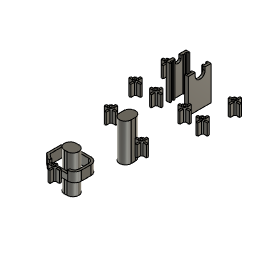
g304base (Autodesk Fusion 360 design; units mm, degrees)
Autodesk Fusion 360 part; units mm, degrees
note: some values were not read from the file. Set by a fixed rule: which sketch regions a step uses.
sketch "草图1" plane through (0, 0, 0) normal (0, 0, 1) x (1, 0, 0)
  circle A0 centre (-11.5, 1.7) radius 1.2
  circle A1 centre (-11.5, 1.7) radius 0.6
  circle A2 centre (11.6, -5.1) radius 0.6
  circle A3 centre (11.6, -5.1) radius 1.2
  circle A4 centre (7.5, 21.6) radius 0.6
  circle A5 centre (7.5, 21.6) radius 1.2
  circle A6 centre (-7.5, 21.6) radius 0.6
  circle A7 centre (-7.5, 21.6) radius 1.2
  circle A8 centre (-17.7, 38) radius 0.6
  circle A9 centre (-17.7, 38) radius 1.2
  circle A10 centre (-17.7, 20.9) radius 0.6
  circle A11 centre (-17.7, 20.9) radius 1.2
  circle A12 centre (17.7, 38) radius 0.6
  circle A13 centre (17.7, 38) radius 1.2
  circle A14 centre (17.7, 20.9) radius 0.6
  circle A15 centre (17.7, 20.9) radius 1.2
  circle A16 centre (0.3, -39.8) radius 0.6
  circle A17 centre (0.3, -39.8) radius 1.2
  dimension "d3" = 2.4
  dimension "d4" = 1.2
  dimension "d10" = 2.4
  dimension "d11" = 1.2
  dimension "d12" = 2.4
  dimension "d13" = 1.2
  dimension "d14" = 2.4
  dimension "d15" = 1.2
  dimension "d16" = 2.4
  dimension "d17" = 1.2
  dimension "d18" = 2.4
  dimension "d19" = 1.2
  dimension "d20" = 2.4
  dimension "d21" = 1.2
  dimension "d22" = 2.4
  dimension "d23" = 1.2
  dimension "d24" = 1.7
  dimension "d25" = 11.5
  dimension "d26" = 5.1
  dimension "d27" = 11.6
  dimension "d28" = 21.6
  dimension "d29" = 7.5
  dimension "d30" = 7.5
  dimension "d32" = 20.9
  dimension "d33" = 17.7
  dimension "d34" = 17.7
  dimension "d35" = 17.1
  dimension "d36" = 2.4
  dimension "d37" = 1.2
  dimension "d38" = 39.8
  dimension "d39" = 0.3
  constraint concentric A0 A1
  constraint concentric A2 A3
  constraint concentric A4 A5
  constraint concentric A6 A7
  constraint concentric A8 A9
  constraint concentric A10 A11
  constraint concentric A12 A13
  constraint concentric A14 A15
  constraint horizontal A4.centre A6.centre
  constraint horizontal A10.centre A14.centre
  constraint vertical A12.centre A14.centre
  constraint vertical A8.centre A10.centre
  constraint horizontal A8.centre A12.centre
  constraint concentric A16 A17
  measures "d3" diameter of A0
  measures "d4" diameter of A1
  measures "d10" diameter of A3
  measures "d11" diameter of A2
  measures "d12" diameter of A5
  measures "d13" diameter of A4
  measures "d14" diameter of A7
  measures "d15" diameter of A6
  measures "d16" diameter of A9
  measures "d17" diameter of A8
  measures "d18" diameter of A11
  measures "d19" diameter of A10
  measures "d20" diameter of A13
  measures "d21" diameter of A12
  measures "d22" diameter of A15
  measures "d23" diameter of A14
  measures "d24" vertical distance of origin A0.centre
  measures "d25" horizontal distance of origin A0.centre
  measures "d26" vertical distance of origin A2.centre
  measures "d27" horizontal distance of origin A2.centre
  measures "d28" vertical distance of origin A4.centre
  measures "d29" horizontal distance of origin A4.centre
  measures "d30" horizontal distance of origin A6.centre
  measures "d32" vertical distance of origin A14.centre
  measures "d33" horizontal distance of origin A14.centre
  measures "d34" horizontal distance of origin A10.centre
  measures "d35" vertical distance of A12.centre A14.centre
  measures "d36" diameter of A17
  measures "d37" diameter of A16
  measures "d38" vertical distance of origin A16.centre
  measures "d39" horizontal distance of origin A16.centre
sketch "草图2" plane through (0, 0, 0) normal (0, 0, 1) x (1, 0, 0)
  circle A0 centre (-11.5, 1.7) radius 1.2
  line L0 (-8.5, 2.2) -> (-14.5, 2.2)
  line L1 (-14.5, 2.2) -> (-14.5, 1.2)
  line L2 (-14.5, 1.2) -> (-8.5, 1.2)
  line L3 (-8.5, 1.2) -> (-8.5, 2.2)
  line L4 (-8.5, 2.2) -> (-14.5, 1.2) construction
  line L5 (-14.5, 2.2) -> (-8.5, 1.2) construction
  line L6 (-11, -1.3) -> (-12, -1.3)
  line L7 (-12, -1.3) -> (-12, 4.7)
  line L8 (-12, 4.7) -> (-11, 4.7)
  line L9 (-11, 4.7) -> (-11, -1.3)
  line L10 (-11, -1.3) -> (-12, 4.7) construction
  line L11 (-12, -1.3) -> (-11, 4.7) construction
  line L12 (11.1, -8.1) -> (11.1, -2.1)
  line L13 (12.1, -2.1) -> (12.1, -8.1)
  line L14 (14.6, -4.6) -> (8.6, -5.6) construction
  line L15 (14.6, -5.6) -> (14.6, -4.6)
  line L16 (11.1, -8.1) -> (12.1, -2.1) construction
  line L17 (8.6, -4.6) -> (14.6, -5.6) construction
  circle A1 centre (11.6, -5.1) radius 1.2
  line L18 (8.6, -5.6) -> (14.6, -5.6)
  line L19 (14.6, -4.6) -> (8.6, -4.6)
  line L20 (11.1, -2.1) -> (12.1, -2.1)
  line L21 (12.1, -8.1) -> (11.1, -8.1)
  line L22 (8.6, -4.6) -> (8.6, -5.6)
  line L23 (12.1, -8.1) -> (11.1, -2.1) construction
  line L24 (-18.2, 17.9) -> (-18.2, 23.9)
  line L25 (-17.2, 23.9) -> (-17.2, 17.9)
  line L26 (-14.7, 21.4) -> (-20.7, 20.4) construction
  line L27 (-14.7, 20.4) -> (-14.7, 21.4)
  line L28 (-18.2, 17.9) -> (-17.2, 23.9) construction
  line L29 (-20.7, 21.4) -> (-14.7, 20.4) construction
  circle A2 centre (-17.7, 20.9) radius 1.2
  line L30 (-20.7, 20.4) -> (-14.7, 20.4)
  line L31 (-14.7, 21.4) -> (-20.7, 21.4)
  line L32 (-18.2, 23.9) -> (-17.2, 23.9)
  line L33 (-17.2, 17.9) -> (-18.2, 17.9)
  line L34 (-20.7, 21.4) -> (-20.7, 20.4)
  line L35 (-17.2, 17.9) -> (-18.2, 23.9) construction
  line L36 (-8, 18.6) -> (-8, 24.6)
  line L37 (-7, 24.6) -> (-7, 18.6)
  line L38 (-4.5, 22.1) -> (-10.5, 21.1) construction
  line L39 (-4.5, 21.1) -> (-4.5, 22.1)
  line L40 (-8, 18.6) -> (-7, 24.6) construction
  line L41 (-10.5, 22.1) -> (-4.5, 21.1) construction
  circle A3 centre (-7.5, 21.6) radius 1.2
  line L42 (-10.5, 21.1) -> (-4.5, 21.1)
  line L43 (-4.5, 22.1) -> (-10.5, 22.1)
  line L44 (-8, 24.6) -> (-7, 24.6)
  line L45 (-7, 18.6) -> (-8, 18.6)
  line L46 (-10.5, 22.1) -> (-10.5, 21.1)
  line L47 (-7, 18.6) -> (-8, 24.6) construction
  line L48 (7, 18.6) -> (7, 24.6)
  line L49 (8, 24.6) -> (8, 18.6)
  line L50 (10.5, 22.1) -> (4.5, 21.1) construction
  line L51 (10.5, 21.1) -> (10.5, 22.1)
  line L52 (7, 18.6) -> (8, 24.6) construction
  line L53 (4.5, 22.1) -> (10.5, 21.1) construction
  circle A4 centre (7.5, 21.6) radius 1.2
  line L54 (4.5, 21.1) -> (10.5, 21.1)
  line L55 (10.5, 22.1) -> (4.5, 22.1)
  line L56 (7, 24.6) -> (8, 24.6)
  line L57 (8, 18.6) -> (7, 18.6)
  line L58 (4.5, 22.1) -> (4.5, 21.1)
  line L59 (8, 18.6) -> (7, 24.6) construction
  line L60 (17.2, 17.9) -> (17.2, 23.9)
  line L61 (18.2, 23.9) -> (18.2, 17.9)
  line L62 (20.7, 21.4) -> (14.7, 20.4) construction
  line L63 (20.7, 20.4) -> (20.7, 21.4)
  line L64 (17.2, 17.9) -> (18.2, 23.9) construction
  line L65 (14.7, 21.4) -> (20.7, 20.4) construction
  circle A5 centre (17.7, 20.9) radius 1.2
  line L66 (14.7, 20.4) -> (20.7, 20.4)
  line L67 (20.7, 21.4) -> (14.7, 21.4)
  line L68 (17.2, 23.9) -> (18.2, 23.9)
  line L69 (18.2, 17.9) -> (17.2, 17.9)
  line L70 (14.7, 21.4) -> (14.7, 20.4)
  line L71 (18.2, 17.9) -> (17.2, 23.9) construction
  line L72 (-18.2, 35) -> (-18.2, 41)
  line L73 (-17.2, 41) -> (-17.2, 35)
  line L74 (-14.7, 38.5) -> (-20.7, 37.5) construction
  line L75 (-14.7, 37.5) -> (-14.7, 38.5)
  line L76 (-18.2, 35) -> (-17.2, 41) construction
  line L77 (-20.7, 38.5) -> (-14.7, 37.5) construction
  circle A6 centre (-17.7, 38) radius 1.2
  line L78 (-20.7, 37.5) -> (-14.7, 37.5)
  line L79 (-14.7, 38.5) -> (-20.7, 38.5)
  line L80 (-18.2, 41) -> (-17.2, 41)
  line L81 (-17.2, 35) -> (-18.2, 35)
  line L82 (-20.7, 38.5) -> (-20.7, 37.5)
  line L83 (-17.2, 35) -> (-18.2, 41) construction
  line L84 (17.2, 35) -> (17.2, 41)
  line L85 (18.2, 41) -> (18.2, 35)
  line L86 (20.7, 38.5) -> (14.7, 37.5) construction
  line L87 (20.7, 37.5) -> (20.7, 38.5)
  line L88 (17.2, 35) -> (18.2, 41) construction
  line L89 (14.7, 38.5) -> (20.7, 37.5) construction
  circle A7 centre (17.7, 38) radius 1.2
  line L90 (14.7, 37.5) -> (20.7, 37.5)
  line L91 (20.7, 38.5) -> (14.7, 38.5)
  line L92 (17.2, 41) -> (18.2, 41)
  line L93 (18.2, 35) -> (17.2, 35)
  line L94 (14.7, 38.5) -> (14.7, 37.5)
  line L95 (18.2, 35) -> (17.2, 41) construction
  line L96 (-0.2, -42.8) -> (-0.2, -36.8)
  line L97 (0.8, -36.8) -> (0.8, -42.8)
  line L98 (3.3, -39.3) -> (-2.7, -40.3) construction
  line L99 (3.3, -40.3) -> (3.3, -39.3)
  line L100 (-0.2, -42.8) -> (0.8, -36.8) construction
  line L101 (-2.7, -39.3) -> (3.3, -40.3) construction
  circle A8 centre (0.3, -39.8) radius 1.2
  line L102 (-2.7, -40.3) -> (3.3, -40.3)
  line L103 (3.3, -39.3) -> (-2.7, -39.3)
  line L104 (-0.2, -36.8) -> (0.8, -36.8)
  line L105 (0.8, -42.8) -> (-0.2, -42.8)
  line L106 (-2.7, -39.3) -> (-2.7, -40.3)
  line L107 (0.8, -42.8) -> (-0.2, -36.8) construction
  point P0 (0.3, -39.8)
  point P1 (11.6, -5.1)
  point P2 (-11.5, 1.7)
  point P3 (-7.5, 21.6)
  point P4 (-17.7, 20.9)
  point P5 (7.5, 21.6)
  point P6 (17.7, 20.9)
  point P7 (17.7, 38)
  point P8 (-17.7, 38)
  point P9 (-11.5, 1.7)
  point P10 (-11.5, 1.7)
  point P11 (11.6, -5.1)
  point P12 (11.6, -5.1)
  point P13 (11.6, -5.1)
  point P14 (-17.7, 20.9)
  point P15 (-17.7, 20.9)
  point P16 (-17.7, 20.9)
  point P17 (-7.5, 21.6)
  point P18 (-7.5, 21.6)
  point P19 (-7.5, 21.6)
  point P20 (7.5, 21.6)
  point P21 (7.5, 21.6)
  point P22 (7.5, 21.6)
  point P23 (17.7, 20.9)
  point P24 (17.7, 20.9)
  point P25 (17.7, 20.9)
  point P26 (-17.7, 38)
  point P27 (-17.7, 38)
  point P28 (-17.7, 38)
  point P29 (17.7, 38)
  point P30 (17.7, 38)
  point P31 (17.7, 38)
  point P32 (0.3, -39.8)
  point P33 (0.3, -39.8)
  point P34 (0.3, -39.8)
  dimension "d42" = 2.4
  dimension "d43" = 6
  dimension "d44" = 1
  dimension "d45" = 1
  dimension "d46" = 6
  dimension "d47" = 2.4
  dimension "d48" = 6
  dimension "d49" = 1
  dimension "d50" = 1
  dimension "d51" = 6
  dimension "d52" = 2.4
  dimension "d53" = 6
  dimension "d54" = 1
  dimension "d55" = 1
  dimension "d56" = 6
  dimension "d57" = 2.4
  dimension "d58" = 6
  dimension "d59" = 1
  dimension "d60" = 1
  dimension "d61" = 6
  dimension "d62" = 2.4
  dimension "d63" = 6
  dimension "d64" = 1
  dimension "d65" = 1
  dimension "d66" = 6
  dimension "d67" = 2.4
  dimension "d68" = 6
  dimension "d69" = 1
  dimension "d70" = 1
  dimension "d71" = 6
  dimension "d72" = 2.4
  dimension "d73" = 6
  dimension "d74" = 1
  dimension "d75" = 1
  dimension "d76" = 6
  dimension "d77" = 2.4
  dimension "d78" = 6
  dimension "d79" = 1
  dimension "d80" = 1
  dimension "d81" = 6
  dimension "d82" = 2.4
  dimension "d83" = 6
  dimension "d84" = 1
  dimension "d85" = 1
  dimension "d86" = 6
  constraint coincident P9 P2
  constraint horizontal L0
  constraint perpendicular L0 L1
  constraint parallel L0 L2
  constraint parallel L1 L3
  constraint coincident L4 P10
  constraint coincident L5 P10
  constraint horizontal L6
  constraint perpendicular L6 L7
  constraint parallel L6 L8
  constraint parallel L7 L9
  constraint coincident L10 P10
  constraint coincident L11 P10
  constraint coincident P10 P9
  constraint coincident P13 P12
  constraint horizontal L19
  constraint perpendicular L19 L22
  constraint parallel L18 L19
  constraint parallel L15 L22
  constraint coincident P13 L14
  constraint coincident P13 L17
  constraint horizontal L21
  constraint perpendicular L12 L21
  constraint parallel L20 L21
  constraint parallel L12 L13
  constraint coincident P13 L23
  constraint coincident P13 L16
  constraint coincident P16 P15
  constraint horizontal L31
  constraint perpendicular L31 L34
  constraint parallel L30 L31
  constraint parallel L27 L34
  constraint coincident P16 L26
  constraint coincident P16 L29
  constraint horizontal L33
  constraint perpendicular L24 L33
  constraint parallel L32 L33
  constraint parallel L24 L25
  constraint coincident P16 L35
  constraint coincident P16 L28
  constraint coincident P19 P18
  constraint horizontal L43
  constraint perpendicular L43 L46
  constraint parallel L42 L43
  constraint parallel L39 L46
  constraint coincident P19 L38
  constraint coincident P19 L41
  constraint horizontal L45
  constraint perpendicular L36 L45
  constraint parallel L44 L45
  constraint parallel L36 L37
  constraint coincident P19 L47
  constraint coincident P19 L40
  constraint coincident P22 P21
  constraint horizontal L55
  constraint perpendicular L55 L58
  constraint parallel L54 L55
  constraint parallel L51 L58
  constraint coincident P22 L50
  constraint coincident P22 L53
  constraint horizontal L57
  constraint perpendicular L48 L57
  constraint parallel L56 L57
  constraint parallel L48 L49
  constraint coincident P22 L59
  constraint coincident P22 L52
  constraint coincident P25 P24
  constraint horizontal L67
  constraint perpendicular L67 L70
  constraint parallel L66 L67
  constraint parallel L63 L70
  constraint coincident P25 L62
  constraint coincident P25 L65
  constraint horizontal L69
  constraint perpendicular L60 L69
  constraint parallel L68 L69
  constraint parallel L60 L61
  constraint coincident P25 L71
  constraint coincident P25 L64
  constraint coincident P28 P27
  constraint horizontal L79
  constraint perpendicular L79 L82
  constraint parallel L78 L79
  constraint parallel L75 L82
  constraint coincident P28 L74
  constraint coincident P28 L77
  constraint horizontal L81
  constraint perpendicular L72 L81
  constraint parallel L80 L81
  constraint parallel L72 L73
  constraint coincident P28 L83
  constraint coincident P28 L76
  constraint coincident P31 P30
  constraint horizontal L91
  constraint perpendicular L91 L94
  constraint parallel L90 L91
  constraint parallel L87 L94
  constraint coincident P31 L86
  constraint coincident P31 L89
  constraint horizontal L93
  constraint perpendicular L84 L93
  constraint parallel L92 L93
  constraint parallel L84 L85
  constraint coincident P31 L95
  constraint coincident P31 L88
  constraint coincident P34 P33
  constraint horizontal L103
  constraint perpendicular L103 L106
  constraint parallel L102 L103
  constraint parallel L99 L106
  constraint coincident P34 L98
  constraint coincident P34 L101
  constraint horizontal L105
  constraint perpendicular L96 L105
  constraint parallel L104 L105
  constraint parallel L96 L97
  constraint coincident P34 L107
  constraint coincident P34 L100
  measures "d42" diameter of A0
  measures "d43" distance of L1.end L2.end
  measures "d44" distance of L0.end L1.end
  measures "d45" distance of L7.end L8.end
  measures "d46" distance of L6.end L7.end
  measures "d47" diameter of A1
  measures "d48" distance of L15.start L14.end
  measures "d49" distance of L14.end L17.start
  measures "d50" distance of L13.start L12.end
  measures "d51" distance of L12.start L12.end
  measures "d52" diameter of A2
  measures "d53" distance of L27.start L26.end
  measures "d54" distance of L26.end L29.start
  measures "d55" distance of L25.start L24.end
  measures "d56" distance of L24.start L24.end
  measures "d57" diameter of A3
  measures "d58" distance of L39.start L38.end
  measures "d59" distance of L38.end L41.start
  measures "d60" distance of L37.start L36.end
  measures "d61" distance of L36.start L36.end
  measures "d62" diameter of A4
  measures "d63" distance of L51.start L50.end
  measures "d64" distance of L50.end L53.start
  measures "d65" distance of L49.start L48.end
  measures "d66" distance of L48.start L48.end
  measures "d67" diameter of A5
  measures "d68" distance of L63.start L62.end
  measures "d69" distance of L62.end L65.start
  measures "d70" distance of L61.start L60.end
  measures "d71" distance of L60.start L60.end
  measures "d72" diameter of A6
  measures "d73" distance of L75.start L74.end
  measures "d74" distance of L74.end L77.start
  measures "d75" distance of L73.start L72.end
  measures "d76" distance of L72.start L72.end
  measures "d77" diameter of A7
  measures "d78" distance of L87.start L86.end
  measures "d79" distance of L86.end L89.start
  measures "d80" distance of L85.start L84.end
  measures "d81" distance of L84.start L84.end
  measures "d82" diameter of A8
  measures "d83" distance of L99.start L98.end
  measures "d84" distance of L98.end L101.start
  measures "d85" distance of L97.start L96.end
  measures "d86" distance of L96.start L96.end
sketch "草图3" plane through (0, 0, 0) normal (0, 0, 1) x (1, 0, 0)
  line L0 (19, 20) -> (16.4, 20)
  line L1 (16.4, 20) -> (16.4, 21.8)
  line L2 (16.4, 21.8) -> (19, 21.8)
  line L3 (19, 21.8) -> (19, 20)
  line L4 (19, 20) -> (16.4, 21.8) construction
  line L5 (16.4, 20) -> (19, 21.8) construction
  line L6 (16.4, 37.1) -> (19, 38.9) construction
  line L7 (19, 37.1) -> (16.4, 37.1)
  line L8 (19, 37.1) -> (16.4, 38.9) construction
  line L9 (16.4, 37.1) -> (16.4, 38.9)
  line L10 (16.4, 38.9) -> (19, 38.9)
  line L11 (19, 38.9) -> (19, 37.1)
  line L12 (-19, 37.1) -> (-16.4, 38.9) construction
  line L13 (-16.4, 37.1) -> (-19, 37.1)
  line L14 (-16.4, 37.1) -> (-19, 38.9) construction
  line L15 (-19, 37.1) -> (-19, 38.9)
  line L16 (-19, 38.9) -> (-16.4, 38.9)
  line L17 (-16.4, 38.9) -> (-16.4, 37.1)
  line L18 (-19, 20) -> (-16.4, 21.8) construction
  line L19 (-16.4, 20) -> (-19, 20)
  line L20 (-16.4, 20) -> (-19, 21.8) construction
  line L21 (-19, 20) -> (-19, 21.8)
  line L22 (-19, 21.8) -> (-16.4, 21.8)
  line L23 (-16.4, 21.8) -> (-16.4, 20)
  point P0 (-17.7, 38)
  point P1 (17.7, 38)
  point P2 (17.7, 20.9)
  point P3 (-17.7, 20.9)
  point P4 (17.7, 20.9)
  point P5 (17.7, 38)
  point P6 (17.7, 38)
  point P7 (-17.7, 38)
  point P8 (-17.7, 38)
  point P9 (-17.7, 20.9)
  point P10 (-17.7, 20.9)
  point P11 (17.7, 38)
  point P12 (-17.7, 38)
  dimension "d92" = 1.8
  dimension "d93" = 2.6
  dimension "d94" = 1.8
  dimension "d95" = 2.6
  dimension "d96" = 1.8
  dimension "d97" = 2.6
  dimension "d98" = 1.8
  dimension "d99" = 2.6
  constraint horizontal L0
  constraint perpendicular L0 L1
  constraint parallel L0 L2
  constraint parallel L1 L3
  constraint coincident L4 P4
  constraint coincident L5 P4
  constraint coincident P4 P2
  constraint horizontal L7
  constraint perpendicular L7 L9
  constraint parallel L7 L10
  constraint parallel L9 L11
  constraint coincident P11 L8
  constraint coincident P11 L6
  constraint coincident P11 P6
  constraint horizontal L13
  constraint perpendicular L13 L15
  constraint parallel L13 L16
  constraint parallel L15 L17
  constraint coincident P12 L14
  constraint coincident P12 L12
  constraint coincident P12 P8
  constraint horizontal L19
  constraint perpendicular L19 L21
  constraint parallel L19 L22
  constraint parallel L21 L23
  constraint coincident P10 L20
  constraint coincident P10 L18
  constraint coincident P10 P9
  measures "d92" distance of L0.start L2.end
  measures "d93" distance of L0.start L0.end
  measures "d94" distance of L7.start L6.end
  measures "d95" distance of L6.start L7.start
  measures "d96" distance of L13.start L12.end
  measures "d97" distance of L12.start L13.start
  measures "d98" distance of L19.start L18.end
  measures "d99" distance of L18.start L19.start
extrude "拉伸5" add sketch "草图1" along normal blind 6.8 contours A0 | A1 | A2 | A3 | A4 | A5 | A6 | A7 | A8 | A9 | A10 | A11 | A12 | A13 | A14 | A15 | A16 | A17 makes body 1 at (1.494, -39.9195, 2.2667) makes body 2 at (8.294, 22.4997, 4.5333) makes body 3 at (18.494, 21.7997, 4.5333) makes body 4 at (-8.3379, 22.459, 4.5333) makes body 5 at (12.794, -5.2195, 2.2667) makes body 6 at (18.894, 37.8805, 2.2667) makes body 7 at (-16.506, 37.8805, 2.2667) makes body 8 at (-16.906, 21.7997, 4.5333) makes body 9 at (-10.306, 1.5805, 2.2667)
extrude "拉伸6" cut sketch "草图3" along normal blind 1 from surface at 6 keep common part bodies 3 6 7 8
extrude "拉伸7" add sketch "草图2" along normal blind 6 contours A0 L0 L2 L9 | A0 L0 L2 L3 | A0 L0 L9 | A0 L2 L9 | A0 L0 L7 L9 | A0 L7 L8 L9 | L0 L2 L7 L9 | A0 L6 L7 L9 | A0 L2 L7 L9 | A0 L0 L7 | A0 L0 L2 L7 | A0 L2 L7 | A0 L0 L1 L2 | L12 L13 A1 L21 | L12 A1 L18 | L12 L13 A1 L18 | L12 A1 L18 L19 | L12 L13 L18 L19 | A1 L18 L19 L22 | L13 A1 L18 | L12 A1 L19 | L12 L13 A1 L19 | L13 A1 L18 L19 | L15 A1 L18 L19 | L12 L13 A1 L20 | L13 A1 L19 | L24 L25 A2 L33 | L24 A2 L30 | L24 L25 A2 L30 | L24 A2 L30 L31 | L24 L25 L30 L31 | A2 L30 L31 L34 | L25 A2 L30 | L24 A2 L31 | L24 L25 A2 L31 | L25 A2 L30 L31 | L27 A2 L30 L31 | L24 L25 A2 L32 | L25 A2 L31 | L36 L37 A3 L45 | L36 A3 L42 | L36 L37 A3 L42 | L36 A3 L42 L43 | L36 L37 L42 L43 | A3 L42 L43 L46 | L37 A3 L42 | L36 A3 L43 | L36 L37 A3 L43 | L37 A3 L42 L43 | L39 A3 L42 L43 | L36 L37 A3 L44 | L37 A3 L43 | L48 L49 A4 L57 | L48 A4 L54 | L48 L49 A4 L54 | L48 A4 L54 L55 | L48 L49 L54 L55 | A4 L54 L55 L58 | L49 A4 L54 | L48 A4 L55 | L48 L49 A4 L55 | L49 A4 L54 L55 | L51 A4 L54 L55 | L48 L49 A4 L56 | L49 A4 L55 | L60 L61 A5 L69 | L60 A5 L66 | L60 L61 A5 L66 | L60 A5 L66 L67 | L60 L61 L66 L67 | A5 L66 L67 L70 | L61 A5 L66 | L60 A5 L67 | L60 L61 A5 L67 | L61 A5 L66 L67 | L63 A5 L66 L67 | L60 L61 A5 L68 | L61 A5 L67 | L72 L73 A6 L81 | L72 A6 L78 | L72 L73 A6 L78 | L72 A6 L78 L79 | L72 L73 L78 L79 | A6 L78 L79 L82 | L73 A6 L78 | L72 A6 L79 | L72 L73 A6 L79 | L73 A6 L78 L79 | L75 A6 L78 L79 | L72 L73 A6 L80 | L73 A6 L79 | L84 L85 A7 L93 | L84 A7 L90 | L84 L85 A7 L90 | L84 A7 L90 L91 | L84 L85 L90 L91 | A7 L90 L91 L94 | L85 A7 L90 | L84 A7 L91 | L84 L85 A7 L91 | L85 A7 L90 L91 | L87 A7 L90 L91 | L84 L85 A7 L92 | L85 A7 L91 | L96 L97 A8 L105 | L96 A8 L102 | L96 L97 A8 L102 | L96 A8 L102 L103 | L96 L97 L102 L103 | A8 L102 L103 L106 | L97 A8 L102 | L96 A8 L103 | L96 L97 A8 L103 | L97 A8 L102 L103 | L99 A8 L102 L103 | L97 A8 L103 bodies 1 2 3 4 5 6 7 8 9
extrude "拉伸8" cut sketch "草图1" along normal blind 100 contours A1 | A2 | A4 | A6 | A8 | A10 | A12 | A14 | A16 bodies 1 2 3 4 5 6 7 8 9
sketch "草图4" plane through (0, 0, 0) normal (0, 0, 1) x (1, 0, 0)
  line L0 (-4.4, 36.2) -> (-6.4, 36.2)
  line L1 (-6.4, 36.2) -> (-6.4, 25.8)
  line L2 (-6.4, 25.8) -> (-4.4, 25.8)
  line L3 (-4.4, 25.8) -> (-4.4, 26.6)
  line L4 (-4.4, 26.6) -> (-5.2, 26.6)
  line L5 (-5.2, 26.6) -> (-5.2, 27.8)
  line L6 (-5.2, 27.8) -> (-4.6, 27.8)
  line L7 (-4.6, 27.8) -> (-4.6, 28.6)
  line L8 (-4.6, 28.6) -> (-5.2, 28.6)
  line L9 (-5.2, 28.6) -> (-5.2, 33.4)
  line L10 (-5.2, 33.4) -> (-4.6, 33.4)
  line L11 (-4.6, 33.4) -> (-4.6, 34.2)
  line L12 (-4.6, 34.2) -> (-5.2, 34.2)
  line L13 (-5.2, 34.2) -> (-5.2, 35.4)
  line L14 (-5.2, 35.4) -> (-4.4, 35.4)
  line L15 (-4.4, 36.2) -> (-4.4, 35.4)
  line L16 (4.4, 24.7) -> (6.4, 24.7)
  line L17 (6.4, 24.7) -> (6.4, 36.7)
  line L18 (6.4, 36.7) -> (4.4, 36.7)
  line L19 (4.4, 36.7) -> (4.4, 35.9)
  line L20 (4.4, 35.9) -> (5.2, 35.9)
  line L21 (5.2, 35.9) -> (5.2, 34.4)
  line L22 (5.2, 34.4) -> (4.6, 34.4)
  line L23 (4.6, 34.4) -> (4.6, 33.6)
  line L24 (4.6, 33.6) -> (5.2, 33.6)
  line L25 (5.2, 33.6) -> (5.2, 28.2)
  line L26 (5.2, 28.2) -> (4.6, 28.2)
  line L27 (4.6, 28.2) -> (4.6, 27.4)
  line L28 (4.6, 27.4) -> (5.2, 27.4)
  line L29 (5.2, 27.4) -> (5.2, 25.5)
  line L30 (5.2, 25.5) -> (4.4, 25.5)
  line L31 (4.4, 25.5) -> (4.4, 24.7)
  dimension "d109" = 25.8
  dimension "d110" = 4.4
  dimension "d111" = 0.8
  dimension "d112" = 0.8
  dimension "d113" = 1.2
  dimension "d114" = 0.8
  dimension "d115" = 2
  dimension "d116" = 4.8
  dimension "d117" = 0.8
  dimension "d119" = 0.6
  dimension "d120" = 10.4
  dimension "d121" = 0.8
  dimension "d122" = 24.7
  dimension "d123" = 4.4
  dimension "d124" = 2
  dimension "d125" = 0.8
  dimension "d126" = 0.8
  dimension "d127" = 1.9
  dimension "d128" = 0.6
  dimension "d129" = 0.8
  dimension "d130" = 5.4
  dimension "d131" = 0.8
  dimension "d132" = 12
  dimension "d133" = 0.8
  constraint horizontal L0
  constraint perpendicular L0 L1
  constraint perpendicular L1 L2
  constraint perpendicular L2 L3
  constraint perpendicular L3 L4
  constraint perpendicular L4 L5
  constraint perpendicular L5 L6
  constraint perpendicular L6 L7
  constraint perpendicular L7 L8
  constraint perpendicular L6 L9
  constraint perpendicular L9 L10
  constraint perpendicular L10 L11
  constraint perpendicular L11 L12
  constraint perpendicular L12 L13
  constraint perpendicular L13 L14
  constraint vertical L15
  constraint collinear L5 L9
  constraint collinear L9 L13
  constraint collinear L7 L11
  constraint collinear L3 L15
  constraint horizontal L16
  constraint perpendicular L16 L17
  constraint perpendicular L17 L18
  constraint perpendicular L18 L19
  constraint perpendicular L19 L20
  constraint perpendicular L20 L21
  constraint perpendicular L19 L22
  constraint perpendicular L22 L23
  constraint perpendicular L23 L24
  constraint perpendicular L24 L25
  constraint perpendicular L23 L26
  constraint perpendicular L24 L27
  constraint perpendicular L27 L28
  constraint perpendicular L28 L29
  constraint perpendicular L29 L30
  constraint vertical L31
  constraint collinear L25 L29
  constraint collinear L23 L27
  constraint collinear L21 L29
  constraint collinear L19 L31
  measures "d109" vertical distance of origin L2.end
  measures "d110" horizontal distance of L2.end origin
  measures "d111" distance of L2.end L3.end
  measures "d112" distance of L3.end L4.end
  measures "d113" distance of L4.end L5.end
  measures "d114" distance of L6.end L7.end
  measures "d115" distance of L1.end L2.end
  measures "d116" distance of L8.end L9.end
  measures "d117" distance of L10.end L11.end
  measures "d119" distance of L7.end L8.end
  measures "d120" distance of L0.end L1.end
  measures "d121" distance of L0.start L14.end
  measures "d122" vertical distance of origin L16.start
  measures "d123" horizontal distance of origin L16.start
  measures "d124" distance of L16.start L16.end
  measures "d125" distance of L16.start L30.end
  measures "d126" distance of L29.end L30.end
  measures "d127" distance of L28.end L29.end
  measures "d128" distance of L27.end L28.end
  measures "d129" distance of L26.end L27.end
  measures "d130" distance of L24.end L25.end
  measures "d131" distance of L22.end L23.end
  measures "d132" distance of L16.end L17.end
  measures "d133" distance of L18.end L19.end
extrude "拉伸9" add sketch "草图4" along normal blind 18 separate body makes body 10 at (-6.4, 32.7333, 6) makes body 11 at (6.4, 28.7, 12)
sketch "草图5" plane through (0, 0, 0) normal (1, 0, 0) x (0, 1, 0)
  circle A0 centre (30.9, 16.8) radius 1.7
  line L0 (32.5, 26.2255) -> (29.3, 26.2255)
  line L1 (29.3, 26.2255) -> (29.3, 16.2255)
  line L2 (29.3, 16.2255) -> (32.5, 16.2255)
  line L3 (32.5, 16.2255) -> (32.5, 26.2255)
  dimension "d136" = 30.9
  dimension "d137" = 3.4
  dimension "d138" = 16.8
  dimension "d139" = 3.2
  dimension "d140" = 10
  constraint horizontal L0
  constraint vertical L1
  constraint horizontal L2
  constraint vertical L3
  constraint coincident A0 L2.end
  constraint coincident A0 L1.end
  measures "d136" horizontal distance of origin A0.centre
  measures "d137" diameter of A0
  measures "d138" vertical distance of origin A0.centre
  measures "d139" distance of L1.end L2.end
  measures "d140" distance of L0.end L1.end
extrude "拉伸10" cut sketch "草图5" against normal up to surface (6.4 mm away) contours A0 L2 | A0 L1 L2 L3 | A0 L0 L1 L3 bodies 10
sketch "草图6" plane through (0, 0, 0) normal (1, 0, 0) x (0, 1, 0)
  circle A0 centre (30.9, 16.3) radius 2.6
  line L0 (28.3, 16.3) -> (33.5, 16.3)
  line L1 (33.5, 16.3) -> (33.5, 26.3)
  line L2 (33.5, 26.3) -> (28.3, 26.3)
  line L3 (28.3, 26.3) -> (28.3, 16.3)
  dimension "d148" = 5.2
  dimension "d149" = 30.9
  dimension "d150" = 16.3
  dimension "d151" = 5.2
  dimension "d152" = 10
  constraint horizontal L0
  constraint vertical L1
  constraint horizontal L2
  constraint vertical L3
  constraint coincident A0 L0.start
  constraint coincident A0 L0.end
  measures "d148" diameter of A0
  measures "d149" horizontal distance of origin A0.centre
  measures "d150" vertical distance of origin A0.centre
  measures "d151" distance of L0.start L0.end
  measures "d152" distance of L0.end L1.end
extrude "拉伸11" cut sketch "草图6" along normal up to surface (6.4 mm away) bodies 11
other "基础网格特征2"
sketch "草图7" plane through (0, 0, 0) normal (0, 0, 1) x (1, 0, 0)
  line L0 (3.1, -2.2) -> (-3.1, -2.2)
  line L1 (-3.1, -2.2) -> (-3.1, 0)
  line L2 (-3.1, 0) -> (3.1, 0)
  line L3 (3.1, 0) -> (3.1, -2.2)
  line L4 (3.1, -2.2) -> (-3.1, 0) construction
  line L5 (-3.1, -2.2) -> (3.1, 0) construction
  circle A0 centre (0, 0) radius 3.1
  circle A1 centre (0, -2.2) radius 3.1
  line L6 (0.7, -27.5) -> (-0.7, -27.5)
  line L7 (-0.7, -27.5) -> (-0.7, -33.7)
  line L8 (-0.7, -33.7) -> (0.7, -33.7)
  line L9 (0.7, -33.7) -> (0.7, -27.5)
  line L10 (0.7, -27.5) -> (-0.7, -33.7) construction
  line L11 (-0.7, -27.5) -> (0.7, -33.7) construction
  circle A2 centre (0.7, -30.6) radius 3.1
  circle A3 centre (-0.7, -30.6) radius 3.1
  line L12 (-5.8, -35.8) -> (4.4, -35.8)
  line L13 (6.8, -33.4) -> (6.8, -28.4)
  line L14 (4.4, -26) -> (-5.8, -26)
  line L15 (-5.8, -26) -> (-7.8, -27.7)
  line L16 (-7.8, -27.7) -> (-7.8, -34.2)
  line L17 (-7.8, -34.2) -> (-5.8, -35.8)
  arc A4 (6.8, -28.4) -> (4.4, -26) centre (4.4, -28.4) ccw
  arc A5 (4.4, -35.8) -> (6.8, -33.4) centre (4.4, -33.4) ccw
  line L18 (4.4, -24.8) -> (-6.2411, -24.8)
  line L19 (-6.2411, -24.8) -> (-9, -27.1451)
  line L20 (-9, -27.1451) -> (-9, -34.7767)
  line L21 (-9, -34.7767) -> (-6.2209, -37)
  line L22 (-6.2209, -37) -> (4.4, -37)
  arc A6 (4.4, -37) -> (8, -33.4) centre (4.4, -33.4) ccw
  line L23 (8, -33.4) -> (8, -28.4)
  arc A7 (8, -28.4) -> (4.4, -24.8) centre (4.4, -28.4) ccw
  point P0 (0, -1.1)
  point P1 (0, -30.6)
  point P2 (6.8, -35.8)
  dimension "d155" = 6.2
  dimension "d156" = 2.2
  dimension "d157" = 1.1
  dimension "d159" = 6.2
  dimension "d160" = 1.4
  dimension "d161" = 30.6
  dimension "d163" = 4.6
  dimension "d164" = 5.2
  dimension "d165" = 7.8
  dimension "d166" = 2.9
  dimension "d167" = 3.6
  dimension "d168" = 5.8
  dimension "d169" = 6.8
  dimension "d170" = 2.4
  dimension "d171" = 2.4
  dimension "d172" = 1.2
  constraint horizontal L0
  constraint perpendicular L0 L1
  constraint parallel L0 L2
  constraint parallel L1 L3
  constraint coincident L4 P0
  constraint coincident L5 P0
  constraint midpoint L2 A0.centre
  constraint coincident L1.end A0
  constraint midpoint L0 A1.centre
  constraint coincident L0.end A1
  constraint horizontal L6
  constraint perpendicular L6 L7
  constraint parallel L6 L8
  constraint parallel L7 L9
  constraint coincident L10 P1
  constraint coincident L11 P1
  constraint midpoint L9 A2.centre
  constraint coincident L6.start A2
  constraint midpoint L7 A3.centre
  constraint coincident L6.end A3
  constraint perpendicular L7 L12
  constraint perpendicular L12 L13
  constraint perpendicular L13 L14
  constraint perpendicular L14 L16
  constraint tangent L14 A4
  constraint tangent L13 A4
  constraint coincident P2 L13
  constraint coincident P2 L12
  constraint tangent L13 A5
  constraint tangent L12 A5
  constraint vertical A0.centre P0
  constraint vertical A0.centre P1
  constraint vertical L12.start L14.end
  measures "d155" distance of L0.start L0.end
  measures "d156" distance of L0.end L1.end
  measures "d157" vertical distance of A0.centre P0
  measures "d159" distance of L6.start L8.end
  measures "d160" distance of L6.start L6.end
  measures "d161" vertical distance of A0.centre P1
  measures "d163" vertical distance of P1 L14.end
  measures "d164" vertical distance of P1 L12.start
  measures "d165" horizontal distance of P1 L15.end
  measures "d166" vertical distance of P1 L15.end
  measures "d167" vertical distance of P1 L16.end
  measures "d168" horizontal distance of P1 L12.start
  measures "d169" horizontal distance of P1 P2
  measures "d170" radius of A4
  measures "d171" radius of A5
extrude "拉伸12" add sketch "草图7" along normal mid plane 20 separate body contours L0 A0 A1 | L3 A0 A1 | L0 A0 A1 | L0 A0 | L0 L2 A0 A1 | L2 A0 A1 | L2 A0 A1 | L0 A0 A1 | L1 A0 A1 | L2 A1 | L2 A0 A1 | L6 A2 A3 | L9 A2 A3 | L9 A2 A3 | L7 A2 A3 | L7 A2 A3 | L9 A3 | L7 L9 A2 A3 | L7 A2 | L8 A2 A3 | L7 A2 A3 | L9 A2 A3 makes body 12 at (-2.3747, 1.9926, 3.3333) makes body 13 at (-3.3041, -32.2819, -3.3333)
extrude "拉伸13" add sketch "草图7" along normal blind 5 separate body contours L18 L19 L20 L21 L22 A6 L23 A7 makes body 14
sketch "草图8" plane through (0, 0, 0) normal (0, 1, 0) x (1, 0, 0)
  line L0 (-5.2, -3.2) -> (4.2, -3.2)
  line L1 (4.2, -3.2) -> (4.2, -8.2)
  line L2 (4.2, -8.2) -> (-5.2, -8.2)
  line L3 (-5.2, -8.2) -> (-5.2, -3.2)
  dimension "d177" = 3.2
  dimension "d178" = 5.2
  dimension "d179" = 4.2
  dimension "d180" = 5
  constraint horizontal L0
  constraint vertical L1
  constraint horizontal L2
  constraint vertical L3
  measures "d177" distance of origin L0
  measures "d178" horizontal distance of origin L0.start
  measures "d179" horizontal distance of origin L0.end
  measures "d180" distance of L0.end L1.end
extrude "拉伸14" cut sketch "草图8" against normal up to surface (1.2 mm away) from surface at -35.8 bodies 14
sketch "草图10" plane through (0, 0, 0) normal (0, 0, 1) x (1, 0, 0)
  circle A0 centre (0, 40) radius 1.2
  circle A1 centre (0, 40) radius 0.6
  point P0 (4.4, 36.7)
  dimension "d184" = 1.2
  dimension "d185" = 2.4
  dimension "d186" = 3.3
  constraint vertical A0.centre origin
  constraint concentric A0 A1
  measures "d184" diameter of A1
  measures "d185" diameter of A0
  measures "d186" vertical distance of A0.centre P0
extrude "拉伸15" add sketch "草图10" along normal blind 3 separate body makes body 15
equation "d3 = d0 + t0"
equation "d4 = d0"
equation "d0 = 1.2 mm" comment "pcb螺丝孔直径"
equation "d1 = 1.8 mm" comment "外壳螺丝孔直径"
equation "t0 = 1.2 mm" comment "螺丝柱厚度"
equation "d10 = d0 + t0"
equation "d11 = d0"
equation "d12 = d0 + t0"
equation "d13 = d0"
equation "d14 = d0 + t0"
equation "d15 = d0"
equation "d16 = d0 + t0"
equation "d17 = d0"
equation "d18 = d0 + t0"
equation "d19 = d0"
equation "d20 = d0 + t0"
equation "d21 = d0"
equation "d22 = d0 + t0"
equation "d23 = d0"
equation "d36 = d0 + t0"
equation "d37 = d0"
equation "d42 = d0 + t0"
equation "d47 = d0 + t0"
equation "d52 = d0 + t0"
equation "d57 = d0 + t0"
equation "d62 = d0 + t0"
equation "d67 = d0 + t0"
equation "d72 = d0 + t0"
equation "d77 = d0 + t0"
equation "d82 = d0 + t0"
equation "d184 = d0"
equation "d185 = d0 + t0"
